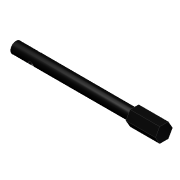
# Autodesk Inventor part: Shovel_RollerDriveAxle
Saved by Autodesk Inventor 2012 (Build 160160000, 160)
## iProperties
Created: 2013-01-30
Part Number: Shovel_RollerDriveAxle
Material: Aluminum-6061-AHC
Document SubType Name: Modeling
Designer: JesseK
Density: 2.71 g/cm^3
Mass: 23.9634 g
Surface Area: 39.7678 cm^2
Volume: 8.84257 cm^3
Author: JesseK
Autodesk Inventor part; units mm, degrees
ref_plane "YZ Plane" through (0, 0, 0) normal (1, 0, 0) x (0, 1, 0)
ref_plane "XZ Plane" through (0, 0, 0) normal (0, 1, 0) x (-1, 0, 0)
ref_plane "XY Plane" through (0, 0, 0) normal (0, 0, 1) x (1, 0, 0)
sketch "Sketch1" plane through (0, 0, 0) normal (1, 0, 0) x (0, 1, 0)
  circle A0 centre (0, 0) radius 4.7625
  dimension "d0" = 9.525
  constraints: 1 centre point, 1 coincident
  measures "d0" diameter of A0
extrude "Extrusion1" add sketch "Sketch1" along normal blind 101.6
sketch "Sketch2" plane through (101.6, 0, 0) normal (1, 0, 0) x (0, 0, -1)
  circle A0 centre (0, 0) radius 4.7625 projected
  line L0 (3.6662, 6.35) -> (7.3323, 0)
  line L1 (7.3323, 0) -> (3.6662, -6.35)
  line L2 (3.6662, -6.35) -> (-3.6662, -6.35)
  line L3 (-3.6662, -6.35) -> (-7.3323, 0)
  line L4 (-7.3323, 0) -> (-3.6662, 6.35)
  line L5 (-3.6662, 6.35) -> (3.6662, 6.35)
  dimension "d3" = 12.7
  constraints: 12 end point, 1 coincident, 1 horizontal, 13 other
  measures "d3" distance between parallel lines of L2 L5
extrude "Extrusion2" add sketch "Sketch2" along normal blind 12.7 contours A0 | L0 L1 L2 L3 L4 L5
sketch "Sketch3" plane through (114.3, 0, -7.3323) normal (0, 0.5, -0.866) x (-1, 0, 0)
  circle A0 centre (76.2, 3.6662) radius 2.4384
  line L0 (12.7, 7.3323) -> (76.2, 7.3323) construction
  line L1 (76.2, 7.3323) -> (76.2, 3.6662) construction
  line L2 (76.2, 3.6662) -> (76.2, 0) construction
  line L3 (76.2, 0) -> (12.7, 0) construction
  point P0 (114.3, 3.6662)
  dimension "d6" = 4.8768
  dimension "d9" = 63.5
  constraints: 8 end point, 2 horizontal, 2 vertical, 1 centre point, 1 collinear
  measures "d6" diameter of A0
  measures "d9" distance of L2.end L3.end
extrude "Extrusion3" cut sketch "Sketch3" against normal through all
body "Solid1"
